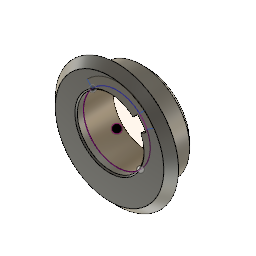
sleeve (Autodesk Fusion 360 design; units mm, degrees)
Autodesk Fusion 360 part; units mm, degrees
sketch "Sketch1" plane through (0, 0, 0) normal (0, 1, 0) x (1, 0, 0)
  circle A0 centre (0, 0) radius 19.5
  circle A1 centre (0, -2) radius 13.5
  line L0 (0, -25.9999) -> (0, 28.2188) construction
  circle A2 centre (14, 6.3554) radius 1.75
  line L1 (-22, 0) -> (22, 0) construction
  circle A3 centre (0, 0) radius 25
  circle A4 centre (14, 6.3554) radius 2.625 construction
  circle A5 centre (-14, 6.3554) radius 1.75
  dimension "d1" = 39
  dimension "d2" = 27
  dimension "d3" = 2
  dimension "d4" = 3.5
  dimension "d5" = 14
  dimension "d7" = 50
  dimension "d9" = 15.375
  measures "d1" diameter of A0
  measures "d2" diameter of A1
  measures "d3" distance of A0.centre
  measures "d4" diameter of A2
  measures "d5" distance of L0
  measures "d7" diameter of A3
  measures "d9" distance of A0.centre
extrude "Extrude2" add sketch "Sketch1" against normal blind 3 contours A0 | A2 | A3 | A5 makes body 1
extrude "Extrude1" add sketch "Sketch1" along normal blind 12 separate body contours A0 makes body 2
chamfer "Chamfer1" distance 3 angle 45 1 edges at (-23.3082, -3, -9.0404) on bodies 1
chamfer "Chamfer2" distance 2 angle 45 1 edges at (-18.1804, 12, 7.0515) on bodies 2
sketch "Sketch7" plane through (0, 0, 0) normal (0, 1, 0) x (1, 0, 0)
  circle A0 centre (0, -2) radius 13.5
  circle A1 centre (0, -2) radius 13.5
  line L0 (-9.871, -11.2095) -> (-12.0169, -13.3068)
  line L1 (14.6969, -9.5) -> (12.1705, -7.842)
  line L2 (9.2095, -11.871) -> (11.2082, -14.109)
  arc A2 (-9.871, -11.2095) -> (9.2095, -11.871) centre (0, -2) ccw
  arc A3 (12.1705, -7.842) -> (9.6243, 7.4669) centre (0, -2) ccw
  arc A4 (11.2082, -14.109) -> (14.6969, -9.5) centre (0, -2) ccw
  arc A5 (-12.0169, -13.3068) -> (11.2082, -14.109) centre (0, -2) ccw
  arc A6 (-9.871, -11.2095) -> (9.2095, -11.871) centre (0, -2) ccw
  dimension "d40" = 5
extrude "Extrude3" cut sketch "Sketch7" against normal through all from surface at 10 contours A0 A1 A2 A3 A6 | A0 A1 L1 L2 A4 bodies 1 2
extrude "Extrude4" cut sketch "Sketch7" along normal blind 5 from surface at 5 contours A0 A1 L0 L2 A2 A5 A6 bodies 2
chamfer "Chamfer5" distance 0.5 angle 45 1 edges at (-10.8781, -3, -5.9948) on bodies 1
